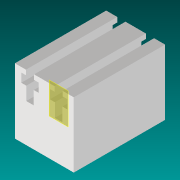
# Autodesk Inventor part: grippershape
Saved by Autodesk Inventor 2020.3 (Build 243373000, 373)
## iProperties
Created: 2020-05-25
Part Number: grippershape
Material: Generic
Document SubType Name: Modeling
Designer: Svend
Density: 1 g/cm^3
Appearance: Default
Author: Svend
Autodesk Inventor part; units mm, degrees
ref_plane "YZ Plane" through (0, 0, 0) normal (1, 0, 0) x (0, 1, 0)
ref_plane "XZ Plane" through (0, 0, 0) normal (0, 1, 0) x (-1, 0, 0)
ref_plane "XY Plane" through (0, 0, 0) normal (0, 0, 1) x (1, 0, 0)
ref_plane "Work Plane1" through (21.95, 0, 0) normal (0, 0, 1) x (1, 0, 0)
sketch "Sketch1" plane through (21.95, 0, 0) normal (0, 0, 1) x (1, 0, 0)
  line L0 (-19.15, -10.8) -> (-24.75, -10.8) projected
  line L1 (-19.15, -0.6) -> (-19.15, -10.8) projected
  line L2 (-15.35, -0.6) -> (-19.15, -0.6) projected
  line L3 (-15.35, 6) -> (-15.35, -0.6) projected
  line L4 (-18.9, 6) -> (-15.35, 6) projected
  line L5 (-18.9, 10.8) -> (-18.9, 6) projected
  line L6 (-25, 10.8) -> (-18.9, 10.8) projected
  line L7 (-25, 6) -> (-25, 10.8) projected
  line L8 (-28.55, 6) -> (-25, 6) projected
  line L9 (-28.55, -0.6) -> (-28.55, 6) projected
  line L10 (-24.75, -0.6) -> (-28.55, -0.6) projected
  line L11 (-24.75, -10.8) -> (-24.75, -0.6) projected
  line L12 (-19, 4.9) -> (-24.9, 4.9) projected
  line L13 (-19, 0.5) -> (-19, 4.9) projected
  line L14 (-24.9, 0.5) -> (-19, 0.5) projected
  line L15 (-24.9, 4.9) -> (-24.9, 0.5) projected
  line L16 (-2.8, -0.6) -> (-6.6, -0.6) projected
  line L17 (-2.8, -10.8) -> (-2.8, -0.6) projected
  line L18 (2.8, -0.6) -> (2.8, -10.8) projected
  line L19 (6.6, -0.6) -> (2.8, -0.6) projected
  line L20 (6.6, 6) -> (6.6, -0.6) projected
  line L21 (3.05, 6) -> (6.6, 6) projected
  line L22 (3.05, 10.8) -> (3.05, 6) projected
  line L23 (-3.05, 10.8) -> (3.05, 10.8) projected
  line L24 (-3.05, 6) -> (-3.05, 10.8) projected
  line L25 (-6.6, 6) -> (-3.05, 6) projected
  line L26 (-6.6, -0.6) -> (-6.6, 6) projected
  line L27 (-33.55, 9.8) -> (11.6, 9.8)
  line L28 (11.6, 9.8) -> (11.6, -40.2)
  line L29 (11.6, -40.2) -> (-33.55, -40.2)
  line L30 (-33.55, -40.2) -> (-33.55, 9.8)
  line L31 (-25.2, 6.2) -> (-28.55, 6.2)
  line L32 (-28.75, 6) -> (-28.75, -0.6)
  line L33 (-28.65, 6.1) -> (-28.75, 6)
  line L34 (-28.55, 6.2) -> (-28.65, 6.1)
  line L35 (-25.2, 10.8) -> (-25.2, 6.2)
  line L36 (-25.1, 10.9) -> (-25.2, 10.8)
  line L37 (-25, 11) -> (-25.1, 10.9)
  line L38 (-18.9, 11) -> (-25, 11)
  line L39 (-18.8, 10.9) -> (-18.9, 11)
  line L40 (-18.7, 10.8) -> (-18.8, 10.9)
  line L41 (-18.7, 6.2) -> (-18.7, 10.8)
  line L42 (-15.35, 6.2) -> (-18.7, 6.2)
  line L43 (-15.25, 6.1) -> (-15.35, 6.2)
  line L44 (-15.15, 6) -> (-15.25, 6.1)
  line L45 (-15.15, -0.6) -> (-15.15, 6)
  line L46 (-15.25, -0.7) -> (-15.15, -0.6)
  line L47 (-15.35, -0.8) -> (-15.25, -0.7)
  line L48 (-18.95, -0.8) -> (-15.35, -0.8)
  line L49 (-18.95, -10.8) -> (-18.95, -0.8)
  line L50 (-19.05, -10.9) -> (-18.95, -10.8)
  line L51 (-19.15, -11) -> (-19.05, -10.9)
  line L52 (-24.75, -11) -> (-19.15, -11)
  line L53 (-24.85, -10.9) -> (-24.75, -11)
  line L54 (-24.95, -10.8) -> (-24.85, -10.9)
  line L55 (-24.95, -0.8) -> (-24.95, -10.8)
  line L56 (-28.55, -0.8) -> (-24.95, -0.8)
  line L57 (-28.65, -0.7) -> (-28.55, -0.8)
  line L58 (-28.75, -0.6) -> (-28.65, -0.7)
  line L59 (-3.25, 10.8) -> (-3.25, 6.2)
  line L60 (-3.15, 10.9) -> (-3.25, 10.8)
  line L61 (-3.05, 11) -> (-3.15, 10.9)
  line L62 (3.05, 11) -> (-3.05, 11)
  line L63 (3.15, 10.9) -> (3.05, 11)
  line L64 (3.25, 10.8) -> (3.15, 10.9)
  line L65 (3.25, 6.2) -> (3.25, 10.8)
  line L66 (6.6, 6.2) -> (3.25, 6.2)
  line L67 (6.7, 6.1) -> (6.6, 6.2)
  line L68 (6.8, 6) -> (6.7, 6.1)
  line L69 (6.8, -0.6) -> (6.8, 6)
  line L70 (6.7, -0.7) -> (6.8, -0.6)
  line L71 (6.6, -0.8) -> (6.7, -0.7)
  line L72 (3, -0.8) -> (6.6, -0.8)
  line L73 (3, -10.8) -> (3, -0.8)
  line L74 (2.8, -11) -> (3, -10.8)
  line L75 (2.8, -10.8) -> (-2.8, -10.8) projected
  line L76 (-2.8, -11) -> (2.8, -11)
  line L77 (-2.9, -10.9) -> (-2.8, -11)
  line L78 (-3, -10.8) -> (-2.9, -10.9)
  line L79 (2.8, -11) -> (2.9, -10.9)
  line L80 (2.9, -10.9) -> (3, -10.8)
  line L81 (-3, -0.8) -> (-3, -10.8)
  line L82 (-6.6, -0.8) -> (-3, -0.8)
  line L83 (-6.7, -0.7) -> (-6.6, -0.8)
  line L84 (-6.8, -0.6) -> (-6.7, -0.7)
  line L85 (-6.8, 6) -> (-6.8, -0.6)
  line L86 (-6.7, 6.1) -> (-6.8, 6)
  line L87 (-6.6, 6.2) -> (-6.7, 6.1)
  line L88 (-3.25, 6.2) -> (-6.6, 6.2)
  line L89 (2.8414, -11.1) -> (-2.8414, -11.1)
  line L90 (-2.8414, -11.1) -> (-2.9707, -10.9707)
  line L91 (-2.9707, -10.9707) -> (-3.1, -10.8414)
  line L92 (-3.1, -10.8414) -> (-3.1, -0.9)
  line L93 (-3.1, -0.9) -> (-6.6414, -0.9)
  line L94 (-6.6414, -0.9) -> (-6.7707, -0.7707)
  line L95 (-6.7707, -0.7707) -> (-6.9, -0.6414)
  line L96 (-6.9, -0.6414) -> (-6.9, 6.0414)
  line L97 (-6.9, 6.0414) -> (-6.7707, 6.1707)
  line L98 (-6.7707, 6.1707) -> (-6.6414, 6.3)
  line L99 (-6.6414, 6.3) -> (-3.35, 6.3)
  line L100 (-3.35, 6.3) -> (-3.35, 10.8414)
  line L101 (-3.35, 10.8414) -> (-3.2207, 10.9707)
  line L102 (-3.2207, 10.9707) -> (-3.0914, 11.1)
  line L103 (-3.0914, 11.1) -> (3.0914, 11.1)
  line L104 (3.0914, 11.1) -> (3.2207, 10.9707)
  line L105 (3.2207, 10.9707) -> (3.35, 10.8414)
  line L106 (3.35, 10.8414) -> (3.35, 6.3)
  line L107 (3.35, 6.3) -> (6.6414, 6.3)
  line L108 (6.6414, 6.3) -> (6.7707, 6.1707)
  line L109 (6.7707, 6.1707) -> (6.9, 6.0414)
  line L110 (6.9, 6.0414) -> (6.9, -0.6414)
  line L111 (6.9, -0.6414) -> (6.7707, -0.7707)
  line L112 (6.7707, -0.7707) -> (6.6414, -0.9)
  line L113 (6.6414, -0.9) -> (3.1, -0.9)
  line L114 (3.1, -0.9) -> (3.1, -10.8414)
  line L115 (-18.85, -0.9) -> (-15.3086, -0.9)
  line L116 (-15.3086, -0.9) -> (-15.1793, -0.7707)
  line L117 (-15.1793, -0.7707) -> (-15.05, -0.6414)
  line L118 (-15.05, -0.6414) -> (-15.05, 6.0414)
  line L119 (-15.05, 6.0414) -> (-15.1793, 6.1707)
  line L120 (-15.1793, 6.1707) -> (-15.3086, 6.3)
  line L121 (-15.3086, 6.3) -> (-18.6, 6.3)
  line L122 (-18.6, 6.3) -> (-18.6, 10.8414)
  line L123 (-18.6, 10.8414) -> (-18.7293, 10.9707)
  line L124 (-18.7293, 10.9707) -> (-18.8586, 11.1)
  line L125 (-18.8586, 11.1) -> (-25.0414, 11.1)
  line L126 (-25.0414, 11.1) -> (-25.1707, 10.9707)
  line L127 (-25.1707, 10.9707) -> (-25.3, 10.8414)
  line L128 (-25.3, 10.8414) -> (-25.3, 6.3)
  line L129 (-25.3, 6.3) -> (-28.5914, 6.3)
  line L130 (-28.5914, 6.3) -> (-28.7207, 6.1707)
  line L131 (-28.7207, 6.1707) -> (-28.85, 6.0414)
  line L132 (-28.85, 6.0414) -> (-28.85, -0.6414)
  line L133 (-28.85, -0.6414) -> (-28.7207, -0.7707)
  line L134 (-28.7207, -0.7707) -> (-28.5914, -0.9)
  line L135 (-28.5914, -0.9) -> (-25.05, -0.9)
  line L136 (-25.05, -0.9) -> (-25.05, -10.8414)
  line L137 (-25.05, -10.8414) -> (-24.9207, -10.9707)
  line L138 (-24.9207, -10.9707) -> (-24.7914, -11.1)
  line L139 (-24.7914, -11.1) -> (-19.1086, -11.1)
  line L140 (-19.1086, -11.1) -> (-18.9793, -10.9707)
  line L141 (-18.9793, -10.9707) -> (-18.85, -10.8414)
  line L142 (-18.85, -10.8414) -> (-18.85, -0.9)
  line L143 (3.1, -10.8414) -> (2.9707, -10.9707)
  line L144 (2.9707, -10.9707) -> (2.8414, -11.1)
  point P0 (-21.95, 0)
  point P1 (-10.975, -0.2)
  point P2 (-10.975, 9.8)
  point P3 (-18.6, 9.8)
  point P4 (-25.3, 9.8)
  point P5 (3.35, 9.8)
  point P6 (-3.35, 9.8)
  dimension "d2" = 11
  dimension "d3" = 4.375
  dimension "d4" = 1
  dimension "d5" = 5
  dimension "d6" = 50
  dimension "d9" = 0.1
  dimension "d10" = 0.1
  dimension "d11" = 0.1
  constraints: 234 end point, 13 horizontal, 12 vertical, 2 parallel, 1 midpoint, 1 perpendicular, 1 vertical alignment, 139 other
  measures "d2" distance from line of point (-10.975, -0.2) L23
  measures "d3" distance from line of L26 point (-10.975, -0.2)
  measures "d4" distance between parallel lines of L23 L27
  measures "d5" distance between parallel lines of L28 L20
  measures "d6" distance of L29.end L27.start
  measures "d9" distance between parallel lines of L69 L110
  measures "d10" distance between parallel lines of L49 L142
  measures "d11" distance between parallel lines of L80 L143
ref_plane "Work Plane2" through (-6.6, -11, -70) normal (0, 0, -1) x (0, 1, 0)
extrude "Extrusion1" add sketch "Sketch1" against normal up to surface (70 mm away) contours L27 L100 L99 L98 L97 L96 L95 L94 L93 L92 L91 L90 L89 L144 L143 L114 L113 L112 L111 L110 L109 L108 L107 L106 L28 L29 L30 L128 L129 L130 L131 L132 L133 L134 L135 L136 L137 L138 L139 L140 L141 L142 L115 L116 L117 L118 L119 L120 L121 L122
body "Solid1"
